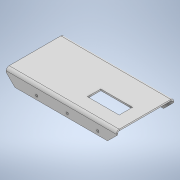
# Autodesk Inventor part: sheetmetalrightside
Saved by Autodesk Inventor 2020.2 (Build 242310000, 310)
## iProperties
Created: 2020-02-05
Part Number: sheetmetalrightside
Material: Generic
Document SubType Name: Sheet Metal
Designer: ColinP
Density: 1 g/cm^3
Sheet Metal Rule: Default
Appearance: Default
Flat Pattern Width: 16.2921 cm
Flat Pattern Length: 22.86 cm
Flat Pattern Area: 372.437 cm^2
Sheet Metal Width: 6.414 in
Sheet Metal Length: 9.000 in
Sheet Metal Area: 57.728 in^2
Author: ColinP
Autodesk Inventor part; units mm, degrees
ref_plane "YZ Plane" through (0, 0, 0) normal (1, 0, 0) x (0, 1, 0)
ref_plane "XZ Plane" through (0, 0, 0) normal (0, 1, 0) x (-1, 0, 0)
ref_plane "XY Plane" through (0, 0, 0) normal (0, 0, 1) x (1, 0, 0)
sketch "Sketch1" plane through (0, 0, 0) normal (0, 0, 1) x (1, 0, 0)
  line L0 (114.3, 63.5) -> (-114.3, 63.5)
  line L1 (-114.3, 63.5) -> (-114.3, -63.5)
  line L2 (-114.3, -63.5) -> (114.3, -63.5)
  line L3 (114.3, -63.5) -> (114.3, 63.5)
  point P0 (0, 0)
  dimension "d0" = 228.6
  dimension "d1" = 127
  measures "d0" distance of L2.end L1.end
  measures "d1" distance of L1.end L0.end
extrude "Plate1" add sketch "Sketch1" along normal blind 3.048
sketch "Sketch2" plane through (0, 0, 3.048) normal (0, 0, 1) x (1, 0, 0)
  line L0 (114.3, 63.5) -> (-114.3, 63.5)
  line L1 (-114.3, 63.5) -> (-96.3395, 81.4605)
  line L2 (-114.3, 63.5) -> (-88.9, 63.5) construction
  line L3 (114.3, 63.5) -> (96.3395, 81.4605)
  line L4 (114.3, 63.5) -> (139.7, 63.5) construction
  line L5 (96.3395, 81.4605) -> (-96.3395, 81.4605)
  line L6 (-114.3, 63.5) -> (-114.3, -63.5)
  line L7 (-114.3, -63.5) -> (-96.3395, -81.4605)
  line L8 (-114.3, -63.5) -> (-88.9, -63.5) construction
  line L9 (-96.3395, -81.4605) -> (96.3395, -81.4605)
  line L10 (-114.3, -63.5) -> (114.3, -63.5)
  line L11 (96.3395, -81.4605) -> (114.3, -63.5)
  point P0 (0, 0)
  dimension "d3" = 25.4
  dimension "d4" = 45
  dimension "d5" = 25.4
  dimension "d6" = 135
  dimension "d7" = 25.4
  dimension "d8" = 45
  measures "d3" distance of L0.end L1.end
  measures "d4" angle of L2 L1
  measures "d5" distance of L0.start L3.end
  measures "d6" angle of L4 L3
  measures "d7" distance of L6.end L7.end
  measures "d8" angle of L7 L8
sheet face with bend "Face2" sketch "Sketch2" thickness 3.048 toward (0, 0, -1) bend radius 3.048
bend "Bend1"
sketch "Sketch3" plane through (0, 0, 3.048) normal (0, 0, 1) x (1, 0, 0)
  line L0 (-114.3, 63.5) -> (-114.3, -63.5) projected
  line L1 (-114.3, 63.5) -> (-114.3, 57.15)
  line L2 (-114.3, 57.15) -> (114.3, 57.15)
  line L3 (114.3, 63.5) -> (114.3, -63.5) projected
  line L4 (114.3, -63.5) -> (114.3, -57.15)
  line L5 (114.3, -57.15) -> (-114.3, -57.15)
  point P0 (0, 0)
  dimension "d14" = 6.35
  dimension "d15" = 6.35
  constraints: 8 end point, 4 point on line, 2 perpendicular
  measures "d14" distance of L0.start L1.end
  measures "d15" distance of L3.end L4.end
fold "Fold1" angle 90 bend radius 3.048 thickness 3.048 k factor 0.44 line from (-114.3, 57.15, 3.048) to (114.3, 57.15, 3.048) line at bend centre moving side (0, 1, 0) folds toward (0, 0, 1)
sketch "Sketch4" plane through (0, 0, 3.048) normal (0, 0, 1) x (1, 0, 0)
  line L0 (-114.3, -63.5) -> (-114.3, 53.7028) projected
  line L1 (-114.3, -63.5) -> (-114.3, -57.15)
  line L2 (-114.3, -57.15) -> (114.3, -57.15)
  line L3 (114.3, -63.5) -> (114.3, 53.7028) projected
  point P0 (0, 0)
  dimension "d22" = 6.35
  constraints: 4 end point, 2 point on line, 1 perpendicular
  measures "d22" distance of L0.start L1.end
fold "Fold2" angle 90 bend radius 3.048 thickness 3.048 k factor 0.44 line from (-114.3, -57.15, 3.048) to (114.3, -57.15, 3.048) line at bend centre moving side (0, 1, 0) folds toward (0, 0, 1)
sketch "Sketch5" plane through (-114.3, -54.5012, 113.5016) normal (0, 1, 0) x (1, 0, 0)
  line L0 (228.6, 0) -> (228.6, -6.096) projected
  line L1 (228.6, 0) -> (228.6, 25.4)
  line L2 (228.6, 0) -> (254, 0) construction
  line L3 (228.6, 25.4) -> (203.2, 25.4)
  line L4 (203.2, 25.4) -> (203.2, 53.34)
  line L5 (203.2, 53.34) -> (137.16, 53.34)
  line L6 (137.16, 53.34) -> (137.16, 25.4)
  line L7 (137.16, 25.4) -> (203.2, 25.4)
  point P0 (114.3, 113.5016)
  dimension "d29" = 25.4
  dimension "d30" = 90
  dimension "d31" = 25.4
  dimension "d32" = 27.94
  dimension "d33" = 66.04
  constraints: 14 end point, 5 perpendicular, 2 vertical, 1 horizontal
  measures "d29" distance of L0.start L1.end
  measures "d30" angle of L2 L1
  measures "d31" distance of L1.end L3.end
  measures "d32" distance of L3.end L4.end
  measures "d33" distance of L4.end L5.end
extrude "Cut1" cut sketch "Sketch5" against normal blind 3.048
sketch "Sketch6" plane through (-96.3395, -81.4605, 116.5496) normal (0, -1, 0) x (1, 0, 0)
  point P0 (96.3395, -116.5496)
sketch "Sketch7" plane through (96.3395, -81.4605, 119.5976) normal (0, 0, -1) x (-1, 0, 0)
  line L0 (192.679, 0) -> (210.6395, 17.9605) projected
  line L1 (210.6395, 17.9605) -> (210.6395, 7.8005)
  line L2 (210.6395, 7.8005) -> (-17.9605, 7.8005)
  line L3 (210.6395, 7.8005) -> (147.1395, 7.8005)
  line L4 (147.1395, 7.8005) -> (83.6395, 7.8005)
  line L5 (83.6395, 7.8005) -> (20.1395, 7.8005)
  line L6 (83.6395, 7.8005) -> (147.1395, 7.8005) construction
  point P0 (96.3395, 81.4605)
  dimension "d36" = 10.16
  dimension "d37" = 228.6
  dimension "d38" = 90
  dimension "d39" = 63.5
  dimension "d40" = 63.5
  dimension "d48" = 63.5
  dimension "d49" = 180
  constraints: 12 end point, 2 collinear, 2 point on line, 1 horizontal, 1 perpendicular, 1 vertical
  measures "d36" distance of L0.end L1.end
  measures "d37" distance of L1.end L2.end
  measures "d38" angle of L1 L2
  measures "d39" distance of L1.end L3.end
  measures "d40" distance of L3.end L4.end
  measures "d48" distance of L4.end L5.end
  measures "d49" angle of L5 L6
hole "Hole1" at (-50.8, -73.66, 119.5976) at (12.7, -73.66, 119.5976) at (76.2, -73.66, 119.5976) direction (0, 0, -1) diameter 4.4958 end through all clearance for "Flat Head Machine Screw (82)" size "#8" standard "Ansi Unified Screw Threads"
equation "\"d2\" = Thickness"
equation "\"d16\" = BendReliefWidth"
equation "\"d17\" = BendReliefDepth"
equation "\"d18\" = MinimumRemnant"
equation "\"d19\" = TransitionRadius"
equation "\"d21\" = BendRadius"
equation "\"d23\" = BendReliefWidth"
equation "\"d24\" = BendReliefDepth"
equation "\"d25\" = MinimumRemnant"
equation "\"d26\" = TransitionRadius"
equation "\"d28\" = BendRadius"
equation "\"d34\" = Thickness"
equation "\"d46\" = Thickness"
equation "\"d9\" = BendRadius"
equation "\"d10\" = BendReliefWidth"
equation "\"d12\" = MinimumRemnant"
equation "\"d11\" = BendReliefDepth"
equation "\"d13\" = TransitionRadius"
equation "\"BendRadius\" = Thickness"
equation "\"BendReliefWidth\" = Thickness"
equation "\"BendReliefDepth\" = 0.5 * Thickness"
equation "\"CornerReliefSize\" = 4 * Thickness"
equation "\"MinimumRemnant\" = 2 * Thickness"
equation "\"TransitionRadius\" = BendRadius"
equation "\"JacobiRadiusSize\" = BendRadius"
equation "\"GapSize\" = Thickness"
equation "\"Thickness\" = 3.048"
body "Solid1"
